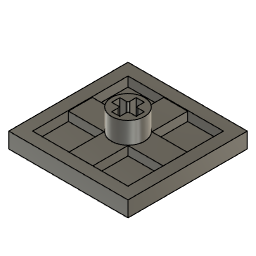
Keycap (Autodesk Fusion 360 design; units mm, degrees)
Autodesk Fusion 360 part; units mm, degrees
sketch "Sketch1" plane through (0, 0, 0) normal (0, 0, 1) x (1, 0, 0)
  circle A0 centre (0, 0) radius 2.77
  line L0 (-10, 10) -> (10, 10)
  line L1 (10, 10) -> (10, -10)
  line L2 (10, -10) -> (-10, -10)
  line L3 (-10, -10) -> (-10, 10)
  line L4 (-10, 0) -> (10, 0) construction
  line L5 (0, 10) -> (0, -10) construction
  line L6 (-0.675, 2.05) -> (0.675, 2.05)
  line L7 (0.675, 2.05) -> (0.675, -2.05)
  line L8 (0.675, -2.05) -> (-0.675, -2.05)
  line L9 (-0.675, -2.05) -> (-0.675, 2.05)
  line L10 (-2.05, 0.675) -> (2.05, 0.675)
  line L11 (2.05, 0.675) -> (2.05, -0.675)
  line L12 (2.05, -0.675) -> (-2.05, -0.675)
  line L13 (-2.05, -0.675) -> (-2.05, 0.675)
  line L14 (-10, 1) -> (10, 1)
  line L15 (10, 1) -> (10, -1)
  line L16 (10, -1) -> (-10, -1)
  line L17 (-10, -1) -> (-10, 1)
  line L18 (1, -10) -> (-1, -10)
  line L19 (-1, -10) -> (-1, 10)
  line L20 (-1, 10) -> (1, 10)
  line L21 (1, 10) -> (1, -10)
  line L22 (-9, 9) -> (9, 9)
  line L23 (9, 9) -> (9, -9)
  line L24 (9, -9) -> (-9, -9)
  line L25 (-9, -9) -> (-9, 9)
  dimension "d1" = 5.54
  dimension "d3" = 20
  dimension "d4" = 20
  dimension "d5" = 4.1
  dimension "d6" = 1.35
  dimension "d7" = 0.675
  dimension "d8" = 2.05
  dimension "d9" = 1.35
  dimension "d10" = 4.1
  dimension "d11" = 2.05
  dimension "d12" = 0.675
  constraint coincident A0.centre origin
  constraint horizontal L0
  constraint vertical L1
  constraint horizontal L2
  constraint vertical L3
  constraint midpoint L3 L4.start
  constraint midpoint L1 L4.end
  constraint midpoint L0 L5.start
  constraint midpoint L2 L5.end
  constraint horizontal L6
  constraint vertical L7
  constraint horizontal L8
  constraint vertical L9
  constraint horizontal L10
  constraint vertical L11
  constraint horizontal L12
  constraint vertical L13
  constraint horizontal L14
  constraint vertical L15
  constraint horizontal L16
  constraint vertical L17
  constraint coincident L1 L15.end
  constraint coincident L3 L14.start
  constraint horizontal L18
  constraint vertical L19
  constraint horizontal L20
  constraint vertical L21
  constraint coincident L0 L19.end
  constraint coincident L2 L18.start
  constraint horizontal L22
  constraint vertical L23
  constraint horizontal L24
  constraint vertical L25
  measures "d1" diameter of A0
  measures "d3" distance of L0.start L2.end
  measures "d4" distance of L0.start L0.end
  measures "d5" distance of L6.start L8.end
  measures "d6" distance of L6.start L6.end
  measures "d7" distance of L5 L7
  measures "d8" distance of L4 L6
  measures "d9" distance of L10.start L12.end
  measures "d10" distance of L10.start L10.end
  measures "d11" distance of L5 L13
  measures "d12" distance of L4 L12
extrude "Extrude1" add sketch "Sketch1" along normal blind 19 contours A0 L10 L11 L12 L14 L16 L21 | A0 L14 L21 | A0 L16 L21 | A0 L6 L7 L9 L14 L19 L21 | L7 L10 L14 L21 | A0 L7 L8 L9 L16 L19 L21 | L7 L12 L16 L21 | A0 L14 L19 | A0 L16 L19 | A0 L10 L12 L13 L14 L16 L19 | L9 L10 L14 L19 | L9 L12 L16 L19
sketch "Sketch2" plane through (0, 0, 0) normal (0, 0, 1) x (1, 0, 0)
  line L0 (-10, 10) -> (10, 10)
  line L1 (10, 10) -> (10, -10)
  line L2 (10, -10) -> (-10, -10)
  line L3 (-10, -10) -> (-10, 10)
  line L4 (-2, 10) -> (2, 10)
  line L5 (2, 10) -> (2, -10)
  line L6 (2, -10) -> (-2, -10)
  line L7 (-2, -10) -> (-2, 10)
  line L8 (-10, 2) -> (10, 2)
  line L9 (10, 2) -> (10, -2)
  line L10 (10, -2) -> (-10, -2)
  line L11 (-10, -2) -> (-10, 2)
  line L12 (-8, 8) -> (8, 8)
  line L13 (8, 8) -> (8, -8)
  line L14 (8, -8) -> (-8, -8)
  line L15 (-8, -8) -> (-8, 8)
  constraint horizontal L0
  constraint vertical L1
  constraint horizontal L2
  constraint vertical L3
  constraint horizontal L4
  constraint vertical L5
  constraint horizontal L6
  constraint vertical L7
  constraint coincident L2 L5.end
  constraint coincident L0 L4.start
  constraint horizontal L8
  constraint vertical L9
  constraint horizontal L10
  constraint vertical L11
  constraint coincident L1 L9.end
  constraint coincident L3 L8.start
  constraint horizontal L12
  constraint vertical L13
  constraint horizontal L14
  constraint vertical L15
extrude "Extrude2" add sketch "Sketch2" along normal blind 6 contours L0 L3 L7 L8 L12 L15 | L0 L4 L5 L7 L12 | L3 L8 L10 L11 L15 | L0 L1 L5 L8 L12 L13 | L5 L7 L8 L12 | L2 L3 L7 L10 L14 L15 | L7 L8 L10 L15 | L5 L7 L8 L10 | L1 L8 L9 L10 L13 | L5 L8 L10 L13 | L5 L7 L10 L14 | L2 L5 L6 L7 L14 | L1 L2 L5 L10 L13 L14
sketch "Sketch3" plane through (0, 0, 0) normal (0, 0, 1) x (1, 0, 0)
  line L0 (-10, -10) -> (10, -10)
  line L1 (10, -10) -> (10, 10)
  line L2 (10, 10) -> (-10, 10)
  line L3 (-10, 10) -> (-10, -10)
  constraint horizontal L0
  constraint vertical L1
  constraint horizontal L2
  constraint vertical L3
extrude "Extrude3" add sketch "Sketch3" against normal blind 1
ref_plane "WorkPlane1" through (0, 0, 6) normal (0, 0, 1) x (1, 0, 0)
sketch "Sketch4" plane through (0, 0, 6) normal (0, 0, 1) x (1, 0, 0)
  line L0 (-10, 10) -> (10, 10)
  line L1 (10, 10) -> (10, -10)
  line L2 (10, -10) -> (-10, -10)
  line L3 (-10, -10) -> (-10, 10)
  line L4 (-8, 8) -> (8, 8)
  line L5 (8, 8) -> (8, -8)
  line L6 (8, -8) -> (-8, -8)
  line L7 (-8, -8) -> (-8, 8)
  constraint horizontal L0
  constraint vertical L1
  constraint horizontal L2
  constraint vertical L3
  constraint horizontal L4
  constraint vertical L5
  constraint horizontal L6
  constraint vertical L7
extrude "Extrude4" add sketch "Sketch4" along normal blind 14
fillet "Fillet1" radius 0.3 4 edges at (0.675, -0.675, 12.5) (-0.675, -0.675, 12.5) (0.675, 0.675, 12.5) (-0.675, 0.675, 12.5)
move_face "MoveFace1" by (0, 0, -18.4) 1 faces at (2.6667, -9.3333, 20)
move_face "MoveFace2" by (0, 0, -12) 1 faces at (1.6852, 1.078, 19)
move_face "MoveFace3" by (0, 0, -4.5) 1 faces at (0.069, -6.2541, 6)
move_face "MoveFace4" by (0, 0, -5) 1 faces at (-0.2595, -0.2494, 6)
move_face "MoveFace5" by (0, 0, -0.5) 1 faces at (-1.6852, 1.078, 7)
move_face "MoveFace6" by (0, 0, -1.4) 1 faces at (-1.6852, 1.078, 6.5)
move_face "MoveFace7" by (0, 0, -0.5) 1 faces at (-0.2595, -0.2494, 1)
named bodies: "Cap"
